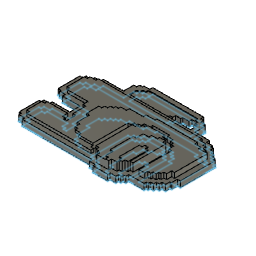
Keychain (Autodesk Fusion 360 design; units mm, degrees)
Autodesk Fusion 360 part; units mm, degrees
sketch "Keychain Among us" plane through (0, 0, 0) normal (0, 0, 1) x (1, 0, 0)
  line L0 (-5, 36) -> (-5, 43)
  line L1 (-5, 43) -> (-3, 43)
  line L2 (-3, 43) -> (-3, 45)
  line L3 (-3, 45) -> (-1, 45)
  line L4 (-1, 45) -> (-1, 46)
  line L5 (-1, 46) -> (3, 46)
  line L6 (3, 48) -> (38, 48)
  line L7 (38, 48) -> (38, 46)
  line L8 (38, 46) -> (40, 46)
  line L9 (40, 46) -> (40, 44)
  line L10 (40, 44) -> (43, 44)
  line L11 (43, 44) -> (43, 43)
  line L12 (43, 43) -> (44, 43)
  line L13 (44, 43) -> (44, 36)
  line L14 (44, 36) -> (54, 36)
  line L15 (54, 36) -> (54, 34)
  line L16 (54, 34) -> (58, 34)
  line L17 (58, 34) -> (58, 32.739)
  line L18 (58, 32.739) -> (60, 32.739)
  line L19 (60, 30.7621) -> (62, 30.7621)
  line L20 (62, 30.7621) -> (62, 29)
  line L21 (62, 29) -> (64, 29)
  line L22 (64, 29) -> (64, 27.4233)
  line L23 (64, 27.4233) -> (66.4467, 27.4233)
  line L24 (66.4467, 27.4233) -> (66.4467, 26)
  line L25 (66.4467, 26) -> (68, 26)
  line L26 (68, 26) -> (68, 2)
  line L27 (68, 2) -> (66, 2)
  line L28 (66, 2) -> (66, -2)
  line L29 (66, -2) -> (65, -2)
  line L30 (65, -2) -> (65, -5.1909)
  line L31 (65, -5.1909) -> (62.4759, -5.1909)
  line L32 (62.4759, -5.1909) -> (62.4759, -7)
  line L33 (62.4759, -7) -> (60.5224, -7)
  line L34 (60.5224, -7) -> (60.5224, -9)
  line L35 (60.5224, -9) -> (58.3587, -9)
  line L36 (58.3587, -9) -> (58.3587, -10.4651)
  line L37 (58.3587, -10.4651) -> (57, -10.4651)
  line L38 (57, -10.4651) -> (57, -12)
  line L39 (57, -12) -> (46.4331, -12)
  line L40 (46.4331, -12) -> (46.4331, -14)
  line L41 (46.4331, -14) -> (44.6217, -14)
  line L42 (44.6217, -14) -> (44.6217, -15.5473)
  line L43 (44.6217, -15.5473) -> (43, -15.5473)
  line L44 (43, -15.5473) -> (43, -17.4243)
  line L45 (43, -17.4243) -> (39, -17.4243)
  line L46 (39, -17.4243) -> (39, -19)
  line L47 (39, -19) -> (29, -19)
  line L48 (29, -19) -> (29, -17.4243)
  line L49 (29, -17.4243) -> (25, -17.4243)
  line L50 (25, -17.4243) -> (25, -15.6805)
  line L51 (25, -15.6805) -> (-23, -15.6805)
  line L52 (-23, -15.6805) -> (-23, -14)
  line L53 (-23, -14) -> (-27, -14)
  line L54 (-27, -14) -> (-27, -12.1957)
  line L55 (-27, -12.1957) -> (-28.5, -12.1957)
  line L56 (-28.5, -12.1957) -> (-28.5, 1.3193)
  line L57 (-28.5, 1.3193) -> (-27, 1.3193)
  line L58 (-27, 1.3193) -> (-27, 3.3222)
  line L59 (-27, 3.3222) -> (-23, 3.3222)
  line L60 (-23, 3.3222) -> (-23, 5)
  line L61 (-23, 5) -> (-11, 5)
  line L62 (-11, 5) -> (-11, 12)
  line L63 (-11, 12) -> (-23, 12)
  line L64 (-23, 12) -> (-23, 14)
  line L65 (-23, 14) -> (-27, 14)
  line L66 (-27, 14) -> (-27, 15)
  line L67 (-27, 15) -> (-29, 15)
  line L68 (-29, 15) -> (-29, 30)
  line L69 (-29, 30) -> (-27, 30)
  line L70 (-27, 30) -> (-27, 32)
  line L71 (-27, 32) -> (-23, 32)
  line L72 (-23, 32) -> (-23, 34)
  line L73 (-23, 34) -> (-19, 34)
  line L74 (-19, 34) -> (-19, 36)
  line L75 (-19, 36) -> (-5, 36)
  line L76 (-1, 36) -> (-1, 41)
  line L77 (-1, 41) -> (1, 41)
  line L78 (1, 41) -> (1, 43)
  line L79 (3, 43) -> (3, 45)
  line L80 (3, 45) -> (37, 45)
  line L81 (37, 43) -> (39, 43)
  line L82 (39, 43) -> (39, 41)
  line L83 (39, 41) -> (41, 41)
  line L84 (41, 41) -> (41, 36)
  line L85 (41, 36) -> (-1, 36)
  line L86 (-18.9747, 32.6312) -> (-18.9747, 31)
  line L87 (-18.9747, 31) -> (-23, 31)
  line L88 (-23, 31) -> (-23, 29)
  line L89 (-23, 29) -> (-25, 29)
  line L90 (-25, 29) -> (-25, 17)
  line L91 (-25, 17) -> (-23, 17)
  line L92 (-23, 17) -> (-23, 15.4917)
  line L93 (-23, 15.4917) -> (-9, 15.4917)
  line L94 (-9, 15.4917) -> (-9, 12)
  line L95 (-9, 12) -> (-7, 12)
  line L96 (-7, 12) -> (-7, 3)
  line L97 (-7, 3) -> (-5, 3)
  line L98 (-5, 3) -> (-5, -3.3505)
  line L99 (-5, -3.3505) -> (-7, -3.3505)
  line L100 (-7, -3.3505) -> (-7, -2)
  line L101 (-7, -2) -> (-9, -2)
  line L102 (-9, -2) -> (-9, 1.5183)
  line L103 (-9, 1.5183) -> (-23, 1.5183)
  line L104 (-23, 1.5183) -> (-23, -0.2408)
  line L105 (-23, -0.2408) -> (-25, -0.2408)
  line L106 (-25, -0.2408) -> (-25, -10.4899)
  line L107 (-25, -10.4899) -> (-23, -10.4899)
  line L108 (-23, -10.4899) -> (-23, -12.5)
  line L109 (-23, -12.5) -> (21, -12.5)
  line L110 (21, -12.5) -> (21, -10.4899)
  line L111 (21, -10.4899) -> (19, -10.4899)
  line L112 (19, -10.4899) -> (19, 15)
  line L113 (19, 15) -> (21, 15)
  line L114 (21, 15) -> (21, 17)
  line L115 (21, 17) -> (23, 17)
  line L116 (23, 17) -> (23, 18)
  line L117 (23, 18) -> (25, 18)
  line L118 (25, 18) -> (25, 20)
  line L119 (25, 20) -> (29, 20)
  line L120 (29, 20) -> (29, 22)
  line L121 (29, 22) -> (40.5686, 22)
  line L122 (40.5686, 22) -> (40.5686, 20.4438)
  line L123 (40.5686, 20.4438) -> (44.5288, 20.4438)
  line L124 (44.5288, 20.4438) -> (44.5288, 18.5)
  line L125 (44.5288, 18.5) -> (46.5, 18.5)
  line L126 (46.5, 18.5) -> (46.5, 17)
  line L127 (46.5, 17) -> (48.5, 17)
  line L128 (48.5, 17) -> (48.5, 13.5)
  line L129 (48.5, 13.5) -> (50.5, 13.5)
  line L130 (50.5, 13.5) -> (50.5, -9)
  line L131 (50.5, -9) -> (54.5326, -9)
  line L132 (54.5326, -9) -> (54.5326, -7)
  line L133 (54.5326, -7) -> (56.6907, -7)
  line L134 (56.6907, -7) -> (56.6907, -5.609)
  line L135 (56.6907, -5.609) -> (59, -5.609)
  line L136 (59, -5.609) -> (59, -3.8218)
  line L137 (59, -3.8218) -> (60.5, -3.8218)
  line L138 (60.5, -3.8218) -> (60.5, -2)
  line L139 (60.5, -2) -> (62.5, -2)
  line L140 (62.5, -2) -> (62.5, 1.5)
  line L141 (62.5, 1.5) -> (64.5, 1.5)
  line L142 (64.5, 1.5) -> (64.5, 24)
  line L143 (64.5, 24) -> (62.5, 24)
  line L144 (62.5, 24) -> (62.5, 26)
  line L145 (62.5, 26) -> (60.5431, 26)
  line L146 (60.5431, 26) -> (60.5431, 27)
  line L147 (60.5431, 27) -> (58.5855, 27)
  line L148 (58.5855, 27) -> (58.5855, 29)
  line L149 (58.5855, 29) -> (56.5, 29)
  line L150 (56.5, 29) -> (56.5, 30.8054)
  line L151 (56.5, 30.8054) -> (52.5, 30.8054)
  line L152 (52.5, 30.8054) -> (52.5, 32.5)
  line L153 (52.5, 32.5) -> (-18.9747, 32.6312)
  line L154 (25, 36) -> (25, 37.6648)
  line L155 (25, 37.6648) -> (27, 37.6648)
  line L156 (27, 37.6648) -> (27, 39.7278)
  line L157 (27, 39.7278) -> (30.5739, 39.7278)
  line L158 (30.5739, 39.7278) -> (30.5739, 41)
  line L159 (30.5739, 41) -> (35, 41)
  line L160 (35, 41) -> (35, 43)
  line L161 (35, 43) -> (37, 43)
  line L162 (19, -9) -> (9, -9)
  line L163 (9, -9) -> (9, -7.2069)
  line L164 (9, -7.2069) -> (5, -7.2069)
  line L165 (5, -7.2069) -> (5, -5.5)
  line L166 (5, -5.5) -> (3, -5.5)
  line L167 (3, -5.5) -> (3, -2)
  line L168 (3, -2) -> (1, -2)
  line L169 (1, -2) -> (1, 6.533)
  line L170 (1, 6.533) -> (-1, 6.533)
  line L171 (-1, 6.533) -> (-1, 15)
  line L172 (-1, 15) -> (1, 15)
  line L173 (1, 15) -> (1, 17)
  line L174 (1, 17) -> (3, 17)
  line L175 (3, 17) -> (3, 19)
  line L176 (3, 19) -> (5, 19)
  line L177 (5, 19) -> (5, 20.468)
  line L178 (5, 20.468) -> (7, 20.468)
  line L179 (7, 20.468) -> (7, 22)
  line L180 (7, 22) -> (11, 22)
  line L181 (11, 22) -> (11, 24)
  line L182 (11, 24) -> (20.478, 24)
  line L183 (20.478, 24) -> (20.478, 26)
  line L184 (20.478, 26) -> (26.6191, 26)
  line L185 (26.6191, 26) -> (26.6191, 27.3324)
  line L186 (26.6191, 27.3324) -> (54.4552, 27.3324)
  line L187 (54.4552, 27.3324) -> (54.4552, 25.5)
  line L188 (54.4552, 25.5) -> (58.5, 25.5)
  line L189 (58.5, 25.5) -> (58.5, 24)
  line L190 (58.5, 24) -> (62.5, 24)
  line L191 (40.5372, 18.7335) -> (29, 18.7335)
  line L192 (29, 18.7335) -> (29, 17)
  line L193 (29, 17) -> (27, 17)
  line L194 (27, 17) -> (27, 15)
  line L195 (27, 15) -> (25, 15)
  line L196 (25, 15) -> (25, 14)
  line L197 (25, 14) -> (23, 14)
  line L198 (23, 14) -> (23, -11)
  line L199 (23, -11) -> (25, -11)
  line L200 (25, -11) -> (25, -13)
  line L201 (25, -13) -> (27, -13)
  line L202 (27, -13) -> (27, -14)
  line L203 (27, -14) -> (28.5711, -14)
  line L204 (28.5711, -14) -> (28.5711, -16)
  line L205 (28.5711, -16) -> (36.7949, -16)
  line L206 (36.7949, -16) -> (36.7949, -14.1381)
  line L207 (36.7949, -14.1381) -> (40.5, -14)
  line L208 (40.5, -14) -> (40.5, -12.5)
  line L209 (40.5, -12.5) -> (42.5, -12.5)
  line L210 (42.5, -12.5) -> (42.5, -10.5)
  line L211 (42.5, -10.5) -> (44.5, -10.5)
  line L212 (44.5, -10.5) -> (44.5, -9)
  line L213 (44.5, -9) -> (46.5, -9)
  line L214 (46.5, -9) -> (46.5, 13.5)
  line L215 (46.5, 13.5) -> (44.5, 13.5)
  line L216 (44.5, 13.5) -> (44.5, 15.5)
  line L217 (44.5, 15.5) -> (42.5, 15.5)
  line L218 (42.5, 15.5) -> (42.5, 17)
  line L219 (42.5, 17) -> (40.5, 17)
  line L220 (40.5, 17) -> (40.5372, 18.7335)
  line L221 (34.6458, -16) -> (34.6458, -14)
  line L222 (34.6458, -14) -> (32.683, -14)
  line L223 (32.683, -14) -> (32.683, -9)
  line L224 (32.683, -9) -> (30.7228, -9)
  line L225 (30.7228, -9) -> (30.7228, 7)
  line L226 (30.7228, 7) -> (32.683, 7)
  line L227 (32.683, 7) -> (32.683, 11.7598)
  line L228 (32.683, 11.7598) -> (36.5, 11.7598)
  line L229 (36.5, 11.7598) -> (36.5, 13.702)
  line L230 (36.5, 13.702) -> (40.5, 13.702)
  line L231 (40.5, 13.702) -> (40.5, 15.2075)
  line L232 (40.5, 15.2075) -> (42.6714, 15.2075)
  line L233 (42.6714, 15.2075) -> (42.5, 15.5)
  line L234 (40.542, 3.1935) -> (40.542, 5)
  line L235 (40.542, 5) -> (42.6807, 5)
  line L236 (42.6807, 5) -> (42.6807, 3.2257)
  line L237 (42.6807, 3.2257) -> (44.5, 3.2257)
  line L238 (44.5, 3.2257) -> (44.5, -9)
  line L239 (40.5, -12.5) -> (40.5, -10.6133)
  line L240 (40.5, -10.6133) -> (38.5507, -10.6133)
  line L241 (38.5507, -10.6133) -> (38.6, 3.2)
  line L242 (40.542, 3.1935) -> (38.6, 3.2)
  line L243 (3, 46) -> (3, 48)
  line L244 (3, 43) -> (1, 43)
  line L245 (37, 45) -> (37, 43)
  line L246 (60, 32.739) -> (60, 30.7621)
  constraint vertical L0
  constraint perpendicular L0 L1
  constraint perpendicular L1 L2
  constraint perpendicular L2 L3
  constraint perpendicular L3 L4
  constraint perpendicular L4 L5
  constraint perpendicular L4 L6
  constraint perpendicular L3 L7
  constraint perpendicular L7 L8
  constraint perpendicular L3 L9
  constraint perpendicular L7 L10
  constraint perpendicular L10 L11
  constraint perpendicular L11 L12
  constraint perpendicular L10 L13
  constraint perpendicular L13 L14
  constraint perpendicular L14 L15
  constraint perpendicular L15 L16
  constraint perpendicular L14 L17
  constraint perpendicular L15 L18
  constraint perpendicular L15 L19
  constraint perpendicular L14 L20
  constraint perpendicular L15 L21
  constraint perpendicular L21 L22
  constraint perpendicular L22 L23
  constraint perpendicular L23 L24
  constraint perpendicular L24 L25
  constraint perpendicular L25 L26
  constraint perpendicular L26 L27
  constraint perpendicular L27 L28
  constraint perpendicular L28 L29
  constraint perpendicular L29 L30
  constraint parallel L28 L32
  constraint perpendicular L31 L32
  constraint perpendicular L32 L33
  constraint perpendicular L33 L34
  constraint perpendicular L34 L35
  constraint perpendicular L35 L36
  constraint perpendicular L36 L37
  constraint perpendicular L35 L38
  constraint perpendicular L36 L39
  constraint perpendicular L35 L40
  constraint perpendicular L40 L41
  constraint perpendicular L35 L42
  constraint perpendicular L42 L43
  constraint perpendicular L43 L44
  constraint perpendicular L44 L45
  constraint perpendicular L43 L46
  constraint perpendicular L44 L47
  constraint perpendicular L47 L48
  constraint perpendicular L48 L49
  constraint perpendicular L47 L50
  constraint perpendicular L48 L51
  constraint perpendicular L51 L52
  constraint perpendicular L52 L53
  constraint perpendicular L53 L54
  constraint perpendicular L54 L55
  constraint perpendicular L55 L56
  constraint perpendicular L56 L57
  constraint perpendicular L57 L58
  constraint perpendicular L56 L59
  constraint perpendicular L57 L60
  constraint perpendicular L60 L61
  constraint perpendicular L61 L62
  constraint perpendicular L62 L63
  constraint perpendicular L63 L64
  constraint perpendicular L64 L65
  constraint perpendicular L65 L66
  constraint perpendicular L66 L67
  constraint perpendicular L65 L68
  constraint perpendicular L68 L69
  constraint perpendicular L65 L70
  constraint perpendicular L68 L71
  constraint perpendicular L71 L72
  constraint perpendicular L68 L73
  constraint perpendicular L71 L74
  constraint perpendicular L0 L75
  constraint vertical L76
  constraint perpendicular L76 L77
  constraint perpendicular L77 L78
  constraint parallel L78 L79
  constraint perpendicular L79 L80
  constraint perpendicular L79 L81
  constraint perpendicular L81 L82
  constraint perpendicular L82 L83
  constraint perpendicular L83 L84
  constraint perpendicular L76 L85
  constraint perpendicular L71 L86
  constraint perpendicular L86 L87
  constraint perpendicular L71 L88
  constraint perpendicular L88 L89
  constraint perpendicular L89 L90
  constraint perpendicular L90 L91
  constraint perpendicular L91 L92
  constraint perpendicular L92 L93
  constraint perpendicular L93 L94
  constraint perpendicular L94 L95
  constraint perpendicular L93 L96
  constraint perpendicular L96 L97
  constraint perpendicular L97 L98
  constraint perpendicular L98 L99
  constraint perpendicular L99 L100
  constraint perpendicular L100 L101
  constraint perpendicular L99 L102
  constraint perpendicular L102 L103
  constraint perpendicular L103 L104
  constraint perpendicular L104 L105
  constraint perpendicular L105 L106
  constraint perpendicular L106 L107
  constraint perpendicular L107 L108
  constraint perpendicular L108 L109
  constraint perpendicular L109 L110
  constraint perpendicular L110 L111
  constraint perpendicular L109 L112
  constraint perpendicular L112 L113
  constraint perpendicular L109 L114
  constraint perpendicular L114 L115
  constraint perpendicular L115 L116
  constraint perpendicular L114 L117
  constraint perpendicular L115 L118
  constraint perpendicular L118 L119
  constraint perpendicular L119 L120
  constraint perpendicular L120 L121
  constraint perpendicular L121 L122
  constraint perpendicular L122 L123
  constraint perpendicular L123 L124
  constraint perpendicular L124 L125
  constraint perpendicular L125 L126
  constraint perpendicular L124 L127
  constraint perpendicular L125 L128
  constraint perpendicular L124 L129
  constraint perpendicular L85 L130
  constraint perpendicular L130 L131
  constraint perpendicular L39 L132
  constraint perpendicular L132 L133
  constraint perpendicular L133 L134
  constraint perpendicular L134 L135
  constraint perpendicular L135 L136
  constraint perpendicular L136 L137
  constraint perpendicular L135 L138
  constraint perpendicular L136 L139
  constraint perpendicular L139 L140
  constraint perpendicular L140 L141
  constraint perpendicular L25 L142
  constraint perpendicular L142 L143
  constraint perpendicular L25 L144
  constraint perpendicular L144 L145
  constraint perpendicular L145 L146
  constraint perpendicular L144 L147
  constraint perpendicular L145 L148
  constraint perpendicular L148 L149
  constraint perpendicular L145 L150
  constraint perpendicular L148 L151
  constraint perpendicular L151 L152
  constraint coincident L85 L154.start
  constraint perpendicular L85 L154
  constraint perpendicular L154 L155
  constraint perpendicular L85 L156
  constraint perpendicular L156 L157
  constraint perpendicular L157 L158
  constraint perpendicular L158 L159
  constraint perpendicular L159 L160
  constraint perpendicular L160 L161
  constraint coincident L112 L162.start
  constraint perpendicular L112 L162
  constraint perpendicular L99 L163
  constraint perpendicular L163 L164
  constraint perpendicular L164 L165
  constraint perpendicular L165 L166
  constraint perpendicular L164 L167
  constraint perpendicular L165 L168
  constraint perpendicular L119 L169
  constraint perpendicular L96 L170
  constraint perpendicular L170 L171
  constraint perpendicular L171 L172
  constraint perpendicular L170 L173
  constraint perpendicular L173 L174
  constraint perpendicular L174 L175
  constraint perpendicular L175 L176
  constraint perpendicular L176 L177
  constraint perpendicular L177 L178
  constraint perpendicular L178 L179
  constraint perpendicular L179 L180
  constraint perpendicular L180 L181
  constraint perpendicular L181 L182
  constraint perpendicular L182 L183
  constraint perpendicular L183 L184
  constraint perpendicular L184 L185
  constraint perpendicular L150 L186
  constraint perpendicular L186 L187
  constraint perpendicular L150 L188
  constraint perpendicular L188 L189
  constraint perpendicular L144 L190
  constraint parallel L121 L191
  constraint perpendicular L191 L192
  constraint perpendicular L192 L193
  constraint perpendicular L193 L194
  constraint perpendicular L194 L195
  constraint perpendicular L195 L196
  constraint perpendicular L196 L197
  constraint perpendicular L197 L198
  constraint perpendicular L198 L199
  constraint perpendicular L199 L200
  constraint perpendicular L200 L201
  constraint perpendicular L201 L202
  constraint perpendicular L202 L203
  constraint perpendicular L203 L204
  constraint perpendicular L202 L205
  constraint perpendicular L203 L206
  constraint perpendicular L203 L208
  constraint perpendicular L208 L209
  constraint perpendicular L203 L210
  constraint perpendicular L210 L211
  constraint perpendicular L211 L212
  constraint perpendicular L210 L213
  constraint perpendicular L39 L214
  constraint perpendicular L214 L215
  constraint perpendicular L39 L216
  constraint perpendicular L216 L217
  constraint perpendicular L217 L218
  constraint perpendicular L218 L219
  constraint coincident L205 L221.start
  constraint perpendicular L205 L221
  constraint perpendicular L221 L222
  constraint perpendicular L205 L223
  constraint perpendicular L221 L224
  constraint perpendicular L205 L225
  constraint perpendicular L225 L226
  constraint perpendicular L226 L227
  constraint perpendicular L227 L228
  constraint perpendicular L228 L229
  constraint perpendicular L229 L230
  constraint perpendicular L230 L231
  constraint perpendicular L231 L232
  constraint parallel L225 L234
  constraint perpendicular L234 L235
  constraint perpendicular L235 L236
  constraint perpendicular L236 L237
  constraint perpendicular L213 L238
  constraint perpendicular L209 L239
  constraint perpendicular L239 L240
  constraint perpendicular L6 L243
  constraint perpendicular L78 L244
  constraint perpendicular L81 L245
  constraint perpendicular L18 L246
extrude "Extrude1" add sketch "Keychain Among us" along normal blind 10 contours L209 L210 L211 L212 L234 L235 L236 L237 L238 L239 L240 L241 L242 makes body 1
extrude "Extrude2" add sketch "Keychain Among us" along normal blind 9.5 contours L205 L206 L207 L208 L213 L214 L215 L216 L217 L221 L222 L223 L224 L225 L226 L227 L228 L229 L230 L231 L232 L233 L234 L235 L236 L237 L238 L239 L240 L241 L242 bodies 1
extrude "Extrude3" add sketch "Keychain Among us" along normal blind 9 contours L191 L192 L193 L194 L195 L196 L197 L198 L199 L200 L201 L202 L203 L204 L205 L218 L219 L220 L221 L222 L223 L224 L225 L226 L227 L228 L229 L230 L231 L232 L233 bodies 1
extrude "Extrude4" add sketch "Keychain Among us" along normal blind 7.5 separate body contours L112 L113 L114 L115 L116 L117 L118 L119 L120 L121 L122 L123 L124 L125 L126 L127 L128 L129 L130 L131 L132 L133 L134 L135 L136 L137 L138 L139 L140 L141 L142 L143 L162 L163 L164 L165 L166 L167 L168 L169 L170 L171 L172 L173 L174 L175 L176 L177 L178 L179 L180 L181 L182 L183 L184 L185 L186 L187 L188 L189 L190 makes body 2
extrude "Extrude5" add sketch "Keychain Among us" along normal blind 6.5 contours L86 L87 L88 L89 L90 L91 L92 L93 L94 L95 L96 L97 L98 L99 L100 L101 L102 L103 L104 L105 L106 L107 L108 L109 L110 L111 L112 L144 L145 L146 L147 L148 L149 L150 L151 L152 L153 L162 L163 L164 L165 L166 L167 L168 L169 L170 L171 L172 L173 L174 L175 L176 L177 L178 L179 L180 L181 L182 L183 L184 L185 L186 L187 L188 L189 L190 bodies 2
extrude "Extrude6" cut 1 faces at (-16.9916, 21.1639, 6.5) along direction (0, 0, -1) blind 0.5 on bodies 2 bodies 2
extrude "Extrude7" add sketch "Keychain Among us" along normal blind 4.5 separate body contours L81 L82 L83 L84 L85 L154 L155 L156 L157 L158 L159 L160 L161 makes body 3
extrude "Extrude8" add sketch "Keychain Among us" along normal blind 3.5 contours L76 L77 L78 L79 L80 L85 L154 L155 L156 L157 L158 L159 L160 L161 L244 L245 bodies 3
extrude "Extrude9" add sketch "Keychain Among us" along normal blind 4 bodies 1 2 3
extrude "Extrude10" cut 1 faces at (35.5246, 38.9093, 4.5) along direction (0, 0, -1) blind 4 on bodies 1 bodies 1
extrude "Extrude11" add sketch "Keychain Among us" against normal blind 1 contours L81 L82 L83 L84 L85 L154 L155 L156 L157 L158 L159 L160 L161 bodies 1
extrude "Extrude12" cut sketch "Keychain Among us" against normal blind 1 contours L81 L82 L83 L84 L85 L154 L155 L156 L157 L158 L159 L160 L161 bodies 1
extrude "Extrude13" cut sketch "Keychain Among us" along normal blind 0.5 contours L81 L82 L83 L84 L85 L154 L155 L156 L157 L158 L159 L160 L161 bodies 1
named bodies: "Keychain Among us"
